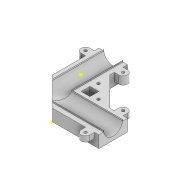
# Autodesk Inventor part: Shaft_Connector_Top_Corner
Saved by Autodesk Inventor 2022 (Build 260153000, 153)
## iProperties
Created: 2022-11-13
Part Number: Shaft_Connector_Top_Corner
Material: Generic
Document SubType Name: Modeling
Designer: MVeszpremi
Density: 1 g/cm^3
Appearance: Default
Author: MVeszpremi
Autodesk Inventor part; units mm, degrees
ref_plane "YZ Plane" through (0, 0, 0) normal (1, 0, 0) x (0, 1, 0)
ref_plane "XZ Plane" through (0, 0, 0) normal (0, 1, 0) x (-1, 0, 0)
ref_plane "XY Plane" through (0, 0, 0) normal (0, 0, 1) x (1, 0, 0)
sketch "Sketch1" plane through (0, 0, 0) normal (0, 1, 0) x (-1, 0, 0)
  line L0 (-32.5, -32.5) -> (32.5, -32.5)
  line L1 (32.5, -32.5) -> (32.5, 32.5)
  line L2 (32.5, 32.5) -> (-32.5, 32.5)
  line L3 (-32.5, 32.5) -> (-32.5, -32.5)
  line L4 (-32.5, -32.5) -> (32.5, 32.5) construction
  line L5 (32.5, -32.5) -> (-32.5, 32.5) construction
  line L6 (-32.5, 0) -> (0, -32.5)
  point P0 (0, 0)
  dimension "d0" = 65
  dimension "d1" = 65
  constraints: 14 end point, 4 midpoint, 2 parallel, 1 horizontal, 1 perpendicular
  measures "d0" distance of L0.end L1.end
  measures "d1" distance of L1.end L2.end
extrude "Extrusion1" add sketch "Sketch1" along normal blind 30 contours L6 L3 L2 L1 L0
sketch "Sketch2" plane through (32.5, 0, 32.5) normal (1, 0, 0) x (0, 0, -1)
  line L0 (0, 0) -> (32.5, 0) projected
  line L1 (0, 30) -> (32.5, 30) projected
  line L2 (0, 0) -> (32.5, 30)
  circle A0 centre (16.25, 15) radius 10.8
  dimension "d5" = 21.6
  constraints: 2 end point, 1 centre point, 1 midpoint
  measures "d5" diameter of A0
extrude "Extrusion2" cut sketch "Sketch2" against normal blind 65.75
sketch "Sketch3" plane through (0, 0, -32.5) normal (0, 0, -1) x (-1, 0, 0)
  line L0 (32.5, 0) -> (32.5, 30) projected
  line L1 (0, 0) -> (32.5, 30)
  circle A0 centre (16.25, 15) radius 10.8
  dimension "d8" = 21.6
  constraints: 2 end point, 1 centre point, 1 midpoint
  measures "d8" diameter of A0
extrude "Extrusion3" cut sketch "Sketch3" against normal blind 65.75
sketch "Sketch4" plane through (0, 0, -32.5) normal (0, 0, -1) x (-1, 0, 0)
  circle A0 centre (16.25, 15) radius 10.8 projected
  line L0 (0, 0) -> (32.5, 0) projected
  line L1 (32.5, 0) -> (32.5, 30) projected
  line L2 (0, 30) -> (32.5, 30) projected
  line L3 (0, 0) -> (0, 30) projected
  point P0 (0, 0)
extrude "Extrusion4" add sketch "Sketch4" along normal blind 20
sketch "Sketch6" plane through (-32.5, 0, 32.5) normal (0, 0, 1) x (1, 0, 0)
  point P0 (32.5, 0)
ref_plane "Work Plane1" through (-32.5, 0, 32.5) normal (0.7071068, 0, 0.7071068) x (0, 1, 0)
mirror "Mirror1" about plane through (-32.5, 0, 32.5) normal (0.7071068, 0, 0.7071068) of "Extrusion4"
sketch "Sketch7" plane through (0, 30, 0) normal (0, 1, 0) x (1, 0, 0)
  line L0 (0, 0) -> (10, 0)
  line L1 (10, 0) -> (10, 10)
  line L2 (10, 10) -> (0, 10)
  line L3 (0, 10) -> (0, 0)
  dimension "d20" = 10
  dimension "d21" = 10
  constraints: 8 end point, 2 parallel, 1 horizontal, 1 perpendicular
  measures "d20" distance of L1.end L2.end
  measures "d21" distance of L0.end L1.end
extrude "Extrusion7" cut sketch "Sketch7" against normal blind 72
sketch "Sketch8" plane through (0, 30, 0) normal (0, 1, 0) x (1, 0, 0)
  point P0 (0, 0)
sketch "Sketch9" plane through (0, 0, 0) normal (0, -1, 0) x (1, 0, 0)
  line L0 (-32.5, 32.5) -> (52.5, 32.5) projected
  line L1 (0, 32.5) -> (-32.5, 0)
  line L2 (-32.5, 32.5) -> (-32.5, -52.5) projected
  line L3 (-16.25, 16.25) -> (-27.05, 27.05) projected
  line L4 (10, -10) -> (0, -10) projected
  line L5 (0, -10) -> (0, 0) projected
  line L6 (0, 0) -> (10, 0) projected
  line L7 (10, 0) -> (10, -10) projected
  line L8 (-32.5, 32.5) -> (52.5, 32.5) projected
  line L9 (-32.5, 32.5) -> (-32.5, -52.5) projected
  line L10 (0, -52.5) -> (-32.5, -52.5) projected
  line L11 (0, -32.5) -> (0, -52.5) projected
  line L12 (32.5, 0) -> (0, -32.5) projected
  line L13 (32.5, 0) -> (52.5, 0) projected
  line L14 (52.5, 0) -> (52.5, 32.5) projected
  constraints: 2 end point, 2 point on line
extrude "Extrusion8" cut sketch "Sketch9" against normal blind 77 contours L0 L1 L2
sketch "Sketch10" plane through (52.5, 0, 0) normal (1, 0, 0) x (0, 0, -1)
  line L0 (-32.5, 0) -> (-32.5, 30) projected
  line L1 (-32.5, 15) -> (70.7005, 15)
  line L2 (-32.5, 18) -> (63.4302, 18)
  line L3 (63.4302, 18) -> (63.4302, 33.0459)
  line L4 (63.4302, 33.0459) -> (-32.5, 33.0459)
  line L5 (-32.5, 33.0459) -> (-32.5, 18)
  line L6 (-32.5, 12) -> (64.9451, 12)
  line L7 (64.9451, 12) -> (64.9451, -20.31)
  line L8 (64.9451, -20.31) -> (-32.5, -20.31)
  line L9 (-32.5, -20.31) -> (-32.5, 12)
  line L10 (32.5, 0) -> (52.5, 0) projected
  line L11 (-32.5, 30) -> (52.5, 30)
  line L12 (52.5, 30) -> (52.5, 0)
  line L13 (52.5, 0) -> (-32.5, 0)
  line L14 (-32.5, 0) -> (-32.5, 30)
  point P0 (0, 0)
  point P1 (52.5, 15)
  dimension "d26" = 3
  dimension "d27" = 3
  constraints: 26 end point, 6 parallel, 4 horizontal, 3 perpendicular, 2 point on line, 1 midpoint
  measures "d26" distance between parallel lines of L1 L2
  measures "d27" distance between parallel lines of L6 L1
extrude "Extrusion9" cut sketch "Sketch10" against normal blind 103.25 contours L0 L2 L12 L1 | L0 L11 L12 L2
sketch "Sketch11" plane through (52.5, 15, 5.45) normal (0, 1, 0) x (1, 0, 0)
  line L0 (-85, 5.45) -> (-85, 57.95) projected
  line L1 (-85, 47.95) -> (-90, 47.95)
  circle A0 centre (-90, 47.95) radius 1.5
  circle A1 centre (-90, 47.95) radius 5
  line L2 (-90, 52.95) -> (-85, 52.95)
  line L3 (-85, 52.95) -> (-85, 42.95)
  line L4 (-85, 42.95) -> (-90, 42.95)
  line L5 (-90, 42.95) -> (-90, 52.95)
  line L6 (-52.5, 57.95) -> (-85, 57.95) projected
  line L7 (-68.75, 57.95) -> (-68.75, 39.1834)
  line L8 (-68.75, -10.8) -> (-79.55, 0) projected
  line L9 (-68.75, -10.8) -> (-16.5653, 41.3847)
  line L10 (-52.5, 47.95) -> (-47.5, 47.95)
  circle A2 centre (-47.5, 47.95) radius 1.5
  circle A3 centre (-47.5, 47.95) radius 5
  line L11 (-47.5, 52.95) -> (-52.5, 52.95)
  line L12 (-52.5, 52.95) -> (-52.5, 42.95)
  line L13 (-52.5, 42.95) -> (-47.5, 42.95)
  line L14 (-47.5, 42.95) -> (-47.5, 52.95)
  line L15 (-10, -27.05) -> (-10, -32.05)
  circle A4 centre (-10, -32.05) radius 1.5
  circle A5 centre (-10, -32.05) radius 5
  line L16 (-5, -32.05) -> (-5, -27.05)
  line L17 (-5, -27.05) -> (-15, -27.05)
  line L18 (-15, -27.05) -> (-15, -32.05)
  line L19 (-15, -32.05) -> (-5, -32.05)
  line L20 (0, 5.45) -> (0, -27.05)
  line L21 (0, -10.8) -> (-18.7666, -10.8)
  line L22 (-10, 5.45) -> (-10, 10.45)
  circle A6 centre (-10, 10.45) radius 1.5
  circle A7 centre (-10, 10.45) radius 5
  line L23 (-5, 10.45) -> (-5, 5.45)
  line L24 (-5, 5.45) -> (-15, 5.45)
  line L25 (-15, 5.45) -> (-15, 10.45)
  line L26 (-15, 10.45) -> (-5, 10.45)
  point P0 (-52.5, 5.45)
  point P1 (-15, -32.05)
  point P2 (-85, 52.95)
  dimension "d30" = 5
  dimension "d31" = 3
  dimension "d32" = 10
  constraints: 48 end point, 28 symmetric about line, 8 centre point, 8 coincident, 8 point on circle, 2 horizontal, 2 parallel, 2 perpendicular, 2 point on line, 1 midpoint, 1 vertical, 6 other
  measures "d30" distance of L1.start L1.end
  measures "d31" diameter of A0
  measures "d32" distance from line of L0.end L1
extrude "Extrusion10" add sketch "Sketch11" against normal blind 7.5 contours L4 A1 L0 | A1 L2 L0 | A1 L5 A0 L1 | L1 A0 L5 A1 | A1 L5 A0 | A3 L14 A2 L10 | L12 L11 A3 | L10 A2 L14 A3 | A3 L13 L12 | A3 L14 A2 | A5 L19 A4 L15 | L17 L16 A5 | L15 A4 L19 A5 | A5 L18 L17 | A5 L19 A4 | A7 L26 A6 L22 | L24 L25 A7 | L22 A6 L26 A7 | A7 L23 L24 | A7 L26 A6
sketch "Sketch12" plane through (52.5, 15, 5.45) normal (0, 1, 0) x (1, 0, 0)
  line L0 (0, 0) -> (-57.95, 0) projected
  line L1 (-57.95, 0) -> (-36.25, 21.7)
  line L2 (-52.5, 37.95) -> (-20, 5.45) projected
  circle A0 centre (-50.45, 22.95) radius 1.5
  line L3 (-57.95, 0) -> (-57.95, 57.95) projected
  line L4 (-42.5, 15.45) -> (-52.5, 15.45) projected
  circle A1 centre (-35, 7.5) radius 1.5
  point P0 (-52.5, 5.45)
  dimension "d35" = 7.5
  dimension "d36" = 7.5
  dimension "d37" = 3
  constraints: 2 centre point, 2 end point, 1 midpoint, 1 symmetric about line, 1 other
  measures "d35" distance from line of L3 A0.centre
  measures "d36" distance from line of L4 A0.centre
  measures "d37" diameter of A0
extrude "Extrusion11" cut sketch "Sketch12" against normal blind 19
sketch "Sketch13" plane through (52.5, 7.5, 5.45) normal (0, -1, 0) x (1, 0, 0)
  circle A0 centre (-90, -47.95) radius 1.5 projected
  line L0 (-93.4641, -47.95) -> (-91.7321, -44.95)
  line L1 (-91.7321, -44.95) -> (-88.2679, -44.95)
  line L2 (-88.2679, -44.95) -> (-86.5359, -47.95)
  line L3 (-86.5359, -47.95) -> (-88.2679, -50.95)
  line L4 (-88.2679, -50.95) -> (-91.7321, -50.95)
  line L5 (-91.7321, -50.95) -> (-93.4641, -47.95)
  line L6 (-85, -42.95) -> (-90, -42.95) projected
  arc A1 (-90, -42.95) -> (-90, -52.95) centre (-90, -47.95) ccw projected
  line L7 (-90, -52.95) -> (-85, -52.95) projected
  line L8 (-85, -42.95) -> (-85, -52.95) projected
  circle A2 centre (-90, -47.95) radius 1.5 projected
  point P0 (-52.5, -5.45)
  dimension "d40" = 6
  constraints: 12 end point, 1 coincident, 13 other
  measures "d40" distance between parallel lines of L1 L4
extrude "Extrusion12" add sketch "Sketch13" along normal blind 3 contours L8 L7 A1 L6
sketch "Sketch14" plane through (52.5, 7.5, 5.45) normal (0, -1, 0) x (1, 0, 0)
  circle A0 centre (-47.5, -47.95) radius 1.5 projected
  line L0 (-50.9641, -47.95) -> (-49.2321, -44.95)
  line L1 (-49.2321, -44.95) -> (-45.7679, -44.95)
  line L2 (-45.7679, -44.95) -> (-44.0359, -47.95)
  line L3 (-44.0359, -47.95) -> (-45.7679, -50.95)
  line L4 (-45.7679, -50.95) -> (-49.2321, -50.95)
  line L5 (-49.2321, -50.95) -> (-50.9641, -47.95)
  line L6 (-47.5, -42.95) -> (-52.5, -42.95) projected
  line L7 (-52.5, -52.95) -> (-52.5, -42.95) projected
  line L8 (-52.5, -52.95) -> (-47.5, -52.95) projected
  arc A1 (-47.5, -52.95) -> (-47.5, -42.95) centre (-47.5, -47.95) ccw projected
  circle A2 centre (-47.5, -47.95) radius 1.5 projected
  point P0 (-52.5, -5.45)
  dimension "d43" = 6
  constraints: 12 end point, 1 coincident, 13 other
  measures "d43" distance between parallel lines of L1 L4
extrude "Extrusion13" add sketch "Sketch14" along normal blind 3 contours A1 L8 L7 L6
sketch "Sketch15" plane through (0, 0, 0) normal (0, -1, 0) x (1, 0, 0)
  circle A0 centre (2.05, -17.5) radius 1.5 projected
  line L0 (-1.4141, -17.5) -> (0.3179, -14.5)
  line L1 (0.3179, -14.5) -> (3.7821, -14.5)
  line L2 (3.7821, -14.5) -> (5.5141, -17.5)
  line L3 (5.5141, -17.5) -> (3.7821, -20.5)
  line L4 (3.7821, -20.5) -> (0.3179, -20.5)
  line L5 (0.3179, -20.5) -> (-1.4141, -17.5)
  circle A1 centre (17.5, -2.05) radius 1.5 projected
  circle A2 centre (17.5, -2.05) radius 5
  point P0 (0, 0)
  dimension "d46" = 6
  dimension "d47" = 10
  constraints: 12 end point, 2 coincident, 1 centre point, 13 other
  measures "d46" distance between parallel lines of L1 L4
  measures "d47" diameter of A2
extrude "Extrusion14" cut sketch "Sketch15" against normal blind 6 contours A0 | L0 L1 L2 L3 L4 L5 | A1 | A2
sketch "Sketch16" plane through (52.5, 15, 5.45) normal (0, 1, 0) x (1, 0, 0)
  circle A0 centre (-50.45, 22.95) radius 1.5 projected
  circle A1 centre (-35, 7.5) radius 1.5 projected
  circle A2 centre (-50.45, 22.95) radius 1.5 projected
  circle A3 centre (-10, 10.45) radius 1.5 projected
  circle A4 centre (-47.5, 47.95) radius 1.5 projected
  line L0 (-57.95, 0) -> (-57.95, 57.95) projected
  line L1 (0, 0) -> (-57.95, 0) projected
  line L2 (0, 5.45) -> (0, 0) projected
  line L3 (-5, 5.45) -> (0, 5.45) projected
  line L4 (-5, 5.45) -> (-5, 10.45) projected
  arc A5 (-5, 10.45) -> (-15, 10.45) centre (-10, 10.45) ccw projected
  line L5 (-15, 10.45) -> (-15, 5.45) projected
  line L6 (-20, 5.45) -> (-15, 5.45) projected
  line L7 (-52.5, 37.95) -> (-20, 5.45) projected
  line L8 (-52.5, 42.95) -> (-52.5, 37.95) projected
  line L9 (-52.5, 42.95) -> (-47.5, 42.95) projected
  arc A6 (-47.5, 42.95) -> (-47.5, 52.95) centre (-47.5, 47.95) ccw projected
  line L10 (-47.5, 52.95) -> (-52.5, 52.95) projected
  line L11 (-52.5, 57.95) -> (-52.5, 52.95) projected
  line L12 (-57.95, 57.95) -> (-52.5, 57.95) projected
  line L13 (-52.5, 5.45) -> (-42.5, 5.45) projected
  line L14 (-52.5, 15.45) -> (-52.5, 5.45) projected
  line L15 (-42.5, 15.45) -> (-52.5, 15.45) projected
  line L16 (-42.5, 5.45) -> (-42.5, 15.45) projected
  circle A7 centre (-90, 47.95) radius 1.5 projected
  line L17 (-79.55, 57.95) -> (-79.55, 0) projected
  line L18 (-85, 57.95) -> (-79.55, 57.95) projected
  line L19 (-85, 52.95) -> (-85, 57.95) projected
  line L20 (-85, 52.95) -> (-90, 52.95) projected
  arc A8 (-90, 52.95) -> (-90, 42.95) centre (-90, 47.95) ccw projected
  line L21 (-90, 42.95) -> (-85, 42.95) projected
  line L22 (-85, 5.45) -> (-85, 42.95) projected
  line L23 (-79.55, 0) -> (-85, 5.45) projected
  circle A9 centre (-10, -32.05) radius 1.5 projected
  line L24 (-57.95, -21.6) -> (0, -21.6) projected
  line L25 (-52.5, -27.05) -> (-57.95, -21.6) projected
  line L26 (-15, -27.05) -> (-52.5, -27.05) projected
  line L27 (-15, -27.05) -> (-15, -32.05) projected
  arc A10 (-15, -32.05) -> (-5, -32.05) centre (-10, -32.05) ccw projected
  line L28 (-5, -32.05) -> (-5, -27.05) projected
  line L29 (0, -27.05) -> (-5, -27.05) projected
  line L30 (0, -21.6) -> (0, -27.05) projected
  point P0 (-52.5, 5.45)
extrude "Extrusion15" cut sketch "Sketch16" against normal blind 1.5
body "Solid1"
